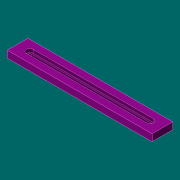
# Autodesk Inventor part: horizontalSupourt
Saved by Autodesk Inventor 2016 (Build 200138000, 138)
## iProperties
Created: 2015-10-27
Part Number: horizontalSupourt
Material: ABS Plastic
Document SubType Name: Modeling
Designer: Sawaiz
Density: 1.06 g/cm^3
Appearance: Smooth - Purple
Author: Sawaiz
Autodesk Inventor part; units mm, degrees
ref_plane "YZ Plane" through (0, 0, 0) normal (1, 0, 0) x (0, 1, 0)
ref_plane "XZ Plane" through (0, 0, 0) normal (0, 1, 0) x (-1, 0, 0)
ref_plane "XY Plane" through (0, 0, 0) normal (0, 0, 1) x (1, 0, 0)
sketch "Sketch1" plane through (0, 0, 0) normal (0, 0, 1) x (1, 0, 0)
  line L0 (-9.525, -66.675) -> (9.525, -66.675)
  line L1 (9.525, -66.675) -> (9.525, 66.675)
  line L2 (9.525, 66.675) -> (-9.525, 66.675)
  line L3 (-9.525, 66.675) -> (-9.525, -66.675)
  line L4 (-9.525, -66.675) -> (9.525, 66.675) construction
  line L5 (9.525, -66.675) -> (-9.525, 66.675) construction
  point P0 (0, 0)
  dimension "d0" = 19.05
  dimension "d1" = 133.35
  constraints: 12 end point, 2 midpoint, 2 parallel, 1 horizontal, 1 perpendicular
  measures "d0" distance of L2.end L1.end
  measures "d1" distance of L1.end L0.end
extrude "Extrusion1" add sketch "Sketch1" along normal blind 6.35
sketch "Sketch4" plane through (0, 0, 6.35) normal (0, 0, 1) x (1, 0, 0)
  line L0 (1.6891, -57.15) -> (-1.6891, -57.15)
  line L1 (-1.6891, -57.15) -> (-1.6891, 57.15)
  line L2 (-1.6891, 57.15) -> (1.6891, 57.15)
  line L3 (1.6891, 57.15) -> (1.6891, -57.15)
  line L4 (1.6891, -57.15) -> (-1.6891, 57.15) construction
  line L5 (-1.6891, -57.15) -> (1.6891, 57.15) construction
  point P0 (0, 0)
  dimension "d16" = 3.3782
  dimension "d17" = 114.3
  constraints: 12 end point, 2 midpoint, 2 parallel, 1 horizontal, 1 perpendicular
  measures "d16" distance of L1.end L2.end
  measures "d17" distance of L0.end L1.end
extrude "Extrusion3" cut sketch "Sketch4" against normal through all
fillet "Fillet2" radius 1.6891 4 edges at (-1.6891, 57.15, 3.175) (1.6891, 57.15, 3.175) (-1.6891, -57.15, 3.175) (1.6891, -57.15, 3.175)
sketch "Sketch5" plane through (0, 0, 6.35) normal (0, 0, 1) x (1, 0, 0)
  line L0 (-3.175, -58.6359) -> (3.175, -58.6359)
  line L1 (3.175, -58.6359) -> (3.175, 58.6359)
  line L2 (3.175, 58.6359) -> (-3.175, 58.6359)
  line L3 (-3.175, 58.6359) -> (-3.175, -58.6359)
  line L4 (-3.175, -58.6359) -> (3.175, 58.6359) construction
  line L5 (3.175, -58.6359) -> (-3.175, 58.6359) construction
  line L6 (1.6891, 55.4609) -> (1.6891, -55.4609) projected
  arc A0 (-1.6891, -55.4609) -> (1.6891, -55.4609) centre (0, -55.4609) ccw projected
  line L7 (-1.6891, -55.4609) -> (-1.6891, 55.4609) projected
  arc A1 (1.6891, 55.4609) -> (-1.6891, 55.4609) centre (0, 55.4609) ccw projected
  line L8 (-9.525, -66.675) -> (9.525, -66.675) projected
  line L9 (9.525, -66.675) -> (9.525, 66.675) projected
  line L10 (9.525, 66.675) -> (-9.525, 66.675) projected
  line L11 (-9.525, 66.675) -> (-9.525, -66.675) projected
  line L12 (-3.175, -58.6359) -> (3.175, -52.2859)
  point P0 (0, 0)
  dimension "d21" = 6.35
  dimension "d31" = 45
  constraints: 14 end point, 3 midpoint, 2 parallel, 1 coincident, 1 horizontal, 1 perpendicular, 1 point on line
  measures "d21" distance of L0.start L0.end
  measures "d31" angle of L0 L12
extrude "Extrusion4" cut sketch "Sketch5" against normal blind 3.175 contours L12 A0 L6 L1 L0 | L3 L2 L1 L12 L6 A1 L7 A0
fillet "Fillet3" radius 3.175 4 edges at (-3.175, -58.6359, 4.7625) (3.175, -58.6359, 4.7625) (3.175, 58.6359, 4.7625) (-3.175, 58.6359, 4.7625)
equation "\"d0\" = sensorHolderDepth"
equation "\"d1\" = width + internalAcrylicThickness"
equation "\"d2\" = acrylicThickness"
equation "\"d17\" = width - 2 * acrylicThickness"
equation "\"d18\" = acrylicThickness"
equation "\"acrylicThickness\" = 6.35"
equation "\"height\" = 127"
equation "\"width\" = 127"
equation "\"depth\" = 273.05"
equation "\"mirrorAngle\" = 5deg"
equation "\"detectorWidth\" = 52"
equation "\"detectorHeight\" = 52"
equation "\"mirrorThickness\" = 3.175"
equation "\"fresnelThickness\" = 0.1"
equation "\"focalLength\" = 76.2"
equation "\"ior\" = 1.49"
equation "\"centerThickness\" = 1.524"
equation "\"fresnelAngle\" = 90deg"
equation "\"fresnelEffectiveDiameter\" = 152.4"
equation "\"mirrorSuppourtWidth\" = 38.1"
equation "\"backGrooveBit\" = 4.8006"
equation "\"detectorOpeningWidth\" = 76.2"
equation "\"detectorOpeningHeight\" = 76.2"
equation "\"sensorHolderSensorHeight\" = 53.975"
equation "\"sensorHolderSensorWidth\" = 53.975"
equation "\"oRingWidth\" = 1.5875"
equation "\"sensorHolderORingID\" = 203.2"
equation "\"sensorHolderFlushORingID\" = 304.8"
equation "\"frontBackORingID\" = 419.1"
equation "\"mirrorGroove\" = 19.05"
equation "\"backMirrorGroove\" = 6.35"
equation "\"fresnelMirrorChamfer\" = 6.35"
equation "\"mirrorGrooveMill\" = 3.175"
equation "\"sensorHolderDepth\" = 19.05"
equation "\"internalAcrylicThicnkess\" = 6.35"
equation "\"frameAcrylicThickness\" = 9.525"
equation "\"internalAcrylicThickness\" = 6.35"
equation "\"aerogelClearence\" = 3.175"
equation "\"backplanePostionOffsett\" = 12.7"
equation "\"backplanePCBWidth\" = 76.2"
equation "\"backplanePCBHeight\" = 76.2"
equation "\"backplaneHoleOffsett\" = 6.35"
equation "\"moduleSlotClearence\" = 0.79375"
body "Solid1"
